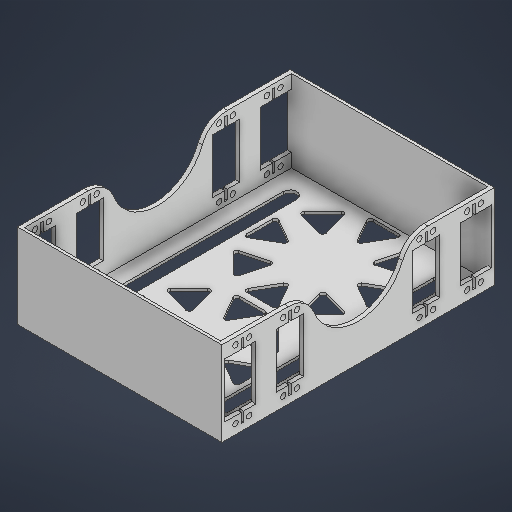
# Autodesk Inventor part: platform
Saved by Autodesk Inventor 2027.1 (Build 311270010, 270A)
## iProperties
Created: 2026-09-04
Part Number: platform
Material: Ogólny
Document SubType Name: Modeling
Designer: User
Density: 1 g/cm^3
Appearance: Domyślna
Author: User
Autodesk Inventor part; units mm, degrees
ref_plane "YZ Plane" through (0, 0, 0) normal (1, 0, 0) x (0, 1, 0)
ref_plane "XZ Plane" through (0, 0, 0) normal (0, 1, 0) x (-1, 0, 0)
ref_plane "XY Plane" through (0, 0, 0) normal (0, 0, 1) x (1, 0, 0)
sketch "Szkic1" plane through (0, 0, 0) normal (0, 1, 0) x (-1, 0, 0)
  line L0 (75, 100) -> (-75, 100)
  line L1 (-75, 100) -> (-75, -100)
  line L2 (-75, -100) -> (75, -100)
  line L3 (75, -100) -> (75, 100)
  line L4 (75, 100) -> (-75, -100) construction
  line L5 (-75, 100) -> (75, -100) construction
  line L6 (70, 95) -> (-70, 95)
  line L7 (-70, 95) -> (-70, -95)
  line L8 (-70, -95) -> (70, -95)
  line L9 (70, -95) -> (70, 95)
  line L10 (70, 95) -> (-70, -95) construction
  line L11 (-70, 95) -> (70, -95) construction
  point P0 (0, 0)
  dimension "d0" = 150
  dimension "d1" = 200
  dimension "d2" = 140
  dimension "d3" = 190
  constraints: 24 end point, 4 midpoint, 4 parallel, 2 horizontal, 2 perpendicular
  measures "d0" distance of L2.end L1.end
  measures "d1" distance of L1.end L0.end
  measures "d2" distance of L8.end L7.end
  measures "d3" distance of L7.end L6.end
extrude "Wyciągnięcie proste1" add sketch "Szkic1" against normal blind 5 contours L3 L2 L1 L0 | L9 L8 L7 L6
extrude "Wyciągnięcie proste2" add sketch "Szkic1" along normal blind 60
sketch "Szkic2" plane through (75, -5, 100) normal (1, 0, 0) x (0, 0, -1)
  line L0 (5, 5) -> (5, 65) construction
  line L1 (0, 65) -> (0, 5) construction
  line L2 (195, 5) -> (5, 5) construction
  line L3 (195, 5) -> (195, 65) construction
  line L4 (5, 5) -> (195, 5) construction
  line L5 (-69.1364, 59.5845) -> (-69.1364, 52.5845)
  line L6 (-69.1364, 52.5845) -> (-70.7364, 52.5845)
  line L7 (-70.7364, 52.5845) -> (-70.7364, 59.5845)
  line L8 (-70.7364, 59.5845) -> (-79.9364, 59.5845)
  line L9 (-79.9364, 59.5845) -> (-79.9364, 99.5845)
  line L10 (-79.9364, 99.5845) -> (-70.7364, 99.5845)
  line L11 (-70.7364, 99.5845) -> (-70.7364, 106.5845)
  line L12 (-70.7364, 106.5845) -> (-69.1364, 106.5845)
  line L13 (-69.1364, 106.5845) -> (-69.1364, 99.5845)
  line L14 (-69.1364, 99.5845) -> (-59.9364, 99.5845)
  line L15 (-59.9364, 99.5845) -> (-59.9364, 59.5845)
  line L16 (-59.9364, 59.5845) -> (-69.1364, 59.5845)
  line L17 (-117.4364, 108.0845) -> (-117.4364, 51.0845)
  line L18 (-117.4364, 51.0845) -> (-57.4364, 51.0845)
  line L19 (-57.4364, 51.0845) -> (-57.4364, 108.0845)
  line L20 (-57.4364, 108.0845) -> (-117.4364, 108.0845)
  circle A0 centre (-64.9364, 54.5845) radius 2
  circle A1 centre (-74.9364, 54.5845) radius 2
  circle A2 centre (-99.9364, 54.5845) radius 2
  circle A3 centre (-109.9364, 54.5845) radius 2
  circle A4 centre (-109.9364, 104.5845) radius 2
  circle A5 centre (-99.9364, 104.5845) radius 2
  circle A6 centre (-74.9364, 104.5845) radius 2
  circle A7 centre (-64.9364, 104.5845) radius 2
  line L21 (-105.7364, 52.5845) -> (-105.7364, 59.5845)
  line L22 (-105.7364, 59.5845) -> (-114.9364, 59.5845)
  line L23 (-114.9364, 59.5845) -> (-114.9364, 99.5845)
  line L24 (-114.9364, 99.5845) -> (-105.7364, 99.5845)
  line L25 (-105.7364, 99.5845) -> (-105.7364, 106.5845)
  line L26 (-105.7364, 106.5845) -> (-104.1364, 106.5845)
  line L27 (-104.1364, 106.5845) -> (-104.1364, 99.5845)
  line L28 (-104.1364, 99.5845) -> (-94.9364, 99.5845)
  line L29 (-94.9364, 99.5845) -> (-94.9364, 59.5845)
  line L30 (-94.9364, 59.5845) -> (-104.1364, 59.5845)
  line L31 (-104.1364, 59.5845) -> (-104.1364, 52.5845)
  line L32 (-104.1364, 52.5845) -> (-105.7364, 52.5845)
  line L33 (0, 35) -> (15, 35)
  line L34 (0, 35) -> (15, 35) construction
  line L35 (-117.4364, 79.5845) -> (-57.4364, 79.5845) construction
  line L36 (-87.4364, 108.0845) -> (-87.4364, 51.0845) construction
  line L37 (195, 35) -> (165, 35)
  circle A8 centre (10, 60) radius 2
  line L38 (15.8, 62) -> (15.8, 55)
  line L39 (14.2, 55) -> (14.2, 62)
  line L40 (14.2, 62) -> (15.8, 62)
  circle A9 centre (20, 60) radius 2
  circle A10 centre (55, 60) radius 2
  line L41 (49.2, 55) -> (49.2, 62)
  line L42 (50.8, 62) -> (50.8, 55)
  line L43 (49.2, 62) -> (50.8, 62)
  circle A11 centre (45, 60) radius 2
  line L44 (5, 55) -> (14.2, 55)
  circle A12 centre (10, 10) radius 2
  line L45 (14.2, 8) -> (14.2, 15)
  line L46 (15.8, 8) -> (14.2, 8)
  line L47 (15.8, 15) -> (15.8, 8)
  line L48 (50.8, 15) -> (50.8, 8)
  line L49 (50.8, 8) -> (49.2, 8)
  line L50 (49.2, 8) -> (49.2, 15)
  circle A13 centre (45, 10) radius 2
  line L51 (60, 15) -> (50.8, 15)
  circle A14 centre (55, 10) radius 2
  line L52 (15.8, 55) -> (25, 55)
  line L53 (40, 55) -> (49.2, 55)
  line L54 (5, 15) -> (5, 55)
  line L55 (14.2, 15) -> (5, 15)
  line L56 (25, 55) -> (25, 15)
  line L57 (50.8, 55) -> (60, 55)
  circle A15 centre (20, 10) radius 2
  line L58 (2.5, 63.5) -> (2.5, 6.5)
  line L59 (62.5, 63.5) -> (2.5, 63.5)
  line L60 (40, 15) -> (40, 55)
  line L61 (60, 55) -> (60, 15)
  line L62 (62.5, 6.5) -> (62.5, 63.5)
  line L63 (49.2, 15) -> (40, 15)
  line L64 (2.5, 6.5) -> (62.5, 6.5)
  line L65 (25, 15) -> (15.8, 15)
  line L66 (2.5, 35) -> (62.5, 35) construction
  line L67 (32.5, 63.5) -> (32.5, 6.5) construction
  line L68 (5, 55) -> (5, 63.5)
  line L69 (5, 15) -> (5, 5)
  point P0 (100, 5)
  point P1 (-104.9364, 79.5845)
  dimension "d8" = 15
  dimension "d10" = 30
  constraints: 134 end point, 16 centre point, 10 midpoint, 2 collinear, 2 horizontal, 2 point on line, 1 vertical
  measures "d8" distance of L33.start L33.end
  measures "d10" distance of L37.start L37.end
extrude "Wyciągnięcie proste3" cut sketch "Szkic2" against normal blind 60 contours L54 L44 L39 L40 L38 L52 L56 L65 L47 L46 L45 L55 | A8 | A9 | A10 | L41 L43 L42 L57 L61 L51 L48 L49 L50 L63 L60 L53 | A11 | A12 | A13 | A14 | A15
pattern_linear "Szyk prostokątny1" count 2 spacing 135 along (0, 0, -1) of "Wyciągnięcie proste3"
mirror "Odbij1" about plane through (0, 0, 0) normal (1, 0, 0) of "Wyciągnięcie proste3", "Szyk prostokątny1"
move faces "Przesuń1" translate (0, 0, 3) faces at (-23.3333, 23.3333, 95)
move faces "Przesuń2" translate (0, 0, -3) faces at (23.3333, 23.3333, -95)
sketch "Szkic3" plane through (75, -5, 100) normal (1, 0, 0) x (0, 0, -1)
  line L0 (0, 65) -> (200, 65) projected
  line L1 (0, 65) -> (200, 65)
  line L2 (100, 65) -> (100, 5)
  circle A0 centre (100, 65) radius 35
  point P0 (135, 65)
  point P1 (65, 65)
  dimension "d22" = 70
  constraints: 4 end point, 1 centre point, 1 coincident, 1 horizontal, 1 midpoint, 1 vertical
  measures "d22" diameter of A0
extrude "Wyciągnięcie proste4" cut sketch "Szkic3" against normal blind 198.25 contours L2 A0 L0 | L0 A0 L2
fillet "Zaokrąglenie1" radius 20 4 edges at (72.5, 60, 35) (72.5, 60, -35) (-72.5, 60, 35) (-72.5, 60, -35)
move faces "Przesuń3" translate (0, 3, 0) faces at (25, -5, 33.3333)
sketch "Szkic4" plane through (0, 0, 0) normal (0, 1, 0) x (1, 0, 0)
  line L0 (-70, 98) -> (-70, -98) projected
  line L1 (70, 98) -> (-70, 98)
  line L2 (-70, 98) -> (-70, -98)
  line L3 (-70, -98) -> (70, -98)
  line L4 (70, -98) -> (70, 98)
  line L5 (70, 98) -> (-70, -98) construction
  line L6 (-70, 98) -> (70, -98) construction
  line L7 (0, 0) -> (0, 25) construction
  line L8 (-1.7321, 22) -> (-11.2583, 5.5)
  line L9 (0, 25) -> (19.0526, 25) construction
  line L10 (1.7321, 22) -> (11.2583, 5.5)
  line L11 (0, 25) -> (19.0526, 25) construction
  line L12 (9.5263, 2.5) -> (-9.5263, 2.5)
  line L13 (0, 25) -> (0, 49) construction
  arc A0 (-11.2583, 5.5) -> (-9.5263, 2.5) centre (-9.5263, 4.5) ccw
  arc A1 (9.5263, 2.5) -> (11.2583, 5.5) centre (9.5263, 4.5) ccw
  arc A2 (1.7321, 22) -> (-1.7321, 22) centre (0, 21) ccw
  arc A3 (22.7983, 10.28) -> (26.1444, 9.3834) centre (24.7302, 10.7977) ccw
  line L14 (39.6166, 22.8556) -> (26.1444, 9.3834)
  line L15 (17.8671, 28.6834) -> (22.7983, 10.28)
  arc A4 (20.3166, 31.1329) -> (17.8671, 28.6834) centre (19.799, 29.201) ccw
  line L16 (34.6482, 14.3518) -> (16.9706, 32.0294) construction
  line L17 (20.3166, 31.1329) -> (38.72, 26.2017)
  line L18 (-84.1457, 34.1508) -> (153.4422, -5.4472) construction
  line L19 (14.8492, 133.1457) -> (54.4472, -104.4422) construction
  arc A5 (39.6166, 22.8556) -> (38.72, 26.2017) centre (38.2023, 24.2698) ccw
  arc A6 (43.5, 37.7417) -> (46.5, 39.4737) centre (44.5, 39.4737) ccw
  line L20 (46.5, 58.5263) -> (46.5, 39.4737)
  line L21 (27, 47.2679) -> (43.5, 37.7417)
  arc A7 (27, 50.7321) -> (27, 47.2679) centre (28, 49) ccw
  line L22 (49, 49) -> (24, 49) construction
  line L23 (27, 50.7321) -> (43.5, 60.2583)
  line L24 (-49, -21) -> (147, 119) construction
  line L25 (-49, 119) -> (147, -21) construction
  arc A8 (46.5, 58.5263) -> (43.5, 60.2583) centre (44.5, 58.5263) ccw
  arc A9 (38.72, 71.7983) -> (39.6166, 75.1444) centre (38.2023, 73.7302) ccw
  line L26 (26.1444, 88.6166) -> (39.6166, 75.1444)
  line L27 (20.3166, 66.8671) -> (38.72, 71.7983)
  arc A10 (17.8671, 69.3166) -> (20.3166, 66.8671) centre (19.799, 68.799) ccw
  line L28 (34.6482, 83.6482) -> (16.9706, 65.9706) construction
  line L29 (17.8671, 69.3166) -> (22.7983, 87.72)
  line L30 (14.8492, -35.1457) -> (54.4472, 202.4422) construction
  line L31 (-84.1457, 63.8492) -> (153.4422, 103.4472) construction
  arc A11 (26.1444, 88.6166) -> (22.7983, 87.72) centre (24.7302, 87.2023) ccw
  arc A12 (11.2583, 92.5) -> (9.5263, 95.5) centre (9.5263, 93.5) ccw
  line L32 (-9.5263, 95.5) -> (9.5263, 95.5)
  line L33 (1.7321, 76) -> (11.2583, 92.5)
  arc A13 (-1.7321, 76) -> (1.7321, 76) centre (0, 77) ccw
  line L34 (0, 98) -> (0, 73) construction
  line L35 (-1.7321, 76) -> (-11.2583, 92.5)
  line L36 (70, 0) -> (-70, 196) construction
  line L37 (-70, 0) -> (70, 196) construction
  arc A14 (-9.5263, 95.5) -> (-11.2583, 92.5) centre (-9.5263, 93.5) ccw
  arc A15 (-22.7983, 87.72) -> (-26.1444, 88.6166) centre (-24.7302, 87.2023) ccw
  line L38 (-39.6166, 75.1444) -> (-26.1444, 88.6166)
  line L39 (-17.8671, 69.3166) -> (-22.7983, 87.72)
  arc A16 (-20.3166, 66.8671) -> (-17.8671, 69.3166) centre (-19.799, 68.799) ccw
  line L40 (-34.6482, 83.6482) -> (-16.9706, 65.9706) construction
  line L41 (-20.3166, 66.8671) -> (-38.72, 71.7983)
  line L42 (84.1457, 63.8492) -> (-153.4422, 103.4472) construction
  line L43 (-14.8492, -35.1457) -> (-54.4472, 202.4422) construction
  arc A17 (-39.6166, 75.1444) -> (-38.72, 71.7983) centre (-38.2023, 73.7302) ccw
  arc A18 (-43.5, 60.2583) -> (-46.5, 58.5263) centre (-44.5, 58.5263) ccw
  line L44 (-46.5, 39.4737) -> (-46.5, 58.5263)
  line L45 (-27, 50.7321) -> (-43.5, 60.2583)
  arc A19 (-27, 47.2679) -> (-27, 50.7321) centre (-28, 49) ccw
  line L46 (-49, 49) -> (-24, 49) construction
  line L47 (-27, 47.2679) -> (-43.5, 37.7417)
  line L48 (49, 119) -> (-147, -21) construction
  line L49 (49, -21) -> (-147, 119) construction
  arc A20 (-46.5, 39.4737) -> (-43.5, 37.7417) centre (-44.5, 39.4737) ccw
  arc A21 (-38.72, 26.2017) -> (-39.6166, 22.8556) centre (-38.2023, 24.2698) ccw
  line L50 (-26.1444, 9.3834) -> (-39.6166, 22.8556)
  line L51 (-20.3166, 31.1329) -> (-38.72, 26.2017)
  arc A22 (-17.8671, 28.6834) -> (-20.3166, 31.1329) centre (-19.799, 29.201) ccw
  line L52 (-34.6482, 14.3518) -> (-16.9706, 32.0294) construction
  line L53 (-17.8671, 28.6834) -> (-22.7983, 10.28)
  line L54 (-14.8492, 133.1457) -> (-54.4472, -104.4422) construction
  line L55 (84.1457, 34.1508) -> (-153.4422, -5.4472) construction
  arc A23 (-26.1444, 9.3834) -> (-22.7983, 10.28) centre (-24.7302, 10.7977) ccw
  line L56 (-70, 0) -> (70, 0) construction
  line L57 (70, -98) -> (-70, 98) construction
  line L58 (-70, -98) -> (70, 98) construction
  line L59 (0, 0) -> (0, -25) construction
  line L60 (-1.7321, -22) -> (-11.2583, -5.5)
  line L61 (0, -25) -> (19.0526, -25) construction
  line L62 (1.7321, -22) -> (11.2583, -5.5)
  line L63 (0, -25) -> (19.0526, -25) construction
  line L64 (9.5263, -2.5) -> (-9.5263, -2.5)
  line L65 (0, -25) -> (0, -49) construction
  arc A24 (-9.5263, -2.5) -> (-11.2583, -5.5) centre (-9.5263, -4.5) ccw
  arc A25 (11.2583, -5.5) -> (9.5263, -2.5) centre (9.5263, -4.5) ccw
  arc A26 (-1.7321, -22) -> (1.7321, -22) centre (0, -21) ccw
  arc A27 (26.1444, -9.3834) -> (22.7983, -10.28) centre (24.7302, -10.7977) ccw
  line L66 (39.6166, -22.8556) -> (26.1444, -9.3834)
  line L67 (17.8671, -28.6834) -> (22.7983, -10.28)
  arc A28 (17.8671, -28.6834) -> (20.3166, -31.1329) centre (19.799, -29.201) ccw
  line L68 (34.6482, -14.3518) -> (16.9706, -32.0294) construction
  line L69 (20.3166, -31.1329) -> (38.72, -26.2017)
  line L70 (-84.1457, -34.1508) -> (153.4422, 5.4472) construction
  line L71 (14.8492, -133.1457) -> (54.4472, 104.4422) construction
  arc A29 (38.72, -26.2017) -> (39.6166, -22.8556) centre (38.2023, -24.2698) ccw
  arc A30 (46.5, -39.4737) -> (43.5, -37.7417) centre (44.5, -39.4737) ccw
  line L72 (46.5, -58.5263) -> (46.5, -39.4737)
  line L73 (27, -47.2679) -> (43.5, -37.7417)
  arc A31 (27, -47.2679) -> (27, -50.7321) centre (28, -49) ccw
  line L74 (49, -49) -> (24, -49) construction
  line L75 (27, -50.7321) -> (43.5, -60.2583)
  line L76 (-49, 21) -> (147, -119) construction
  line L77 (-49, -119) -> (147, 21) construction
  arc A32 (43.5, -60.2583) -> (46.5, -58.5263) centre (44.5, -58.5263) ccw
  arc A33 (39.6166, -75.1444) -> (38.72, -71.7983) centre (38.2023, -73.7302) ccw
  line L78 (26.1444, -88.6166) -> (39.6166, -75.1444)
  line L79 (20.3166, -66.8671) -> (38.72, -71.7983)
  arc A34 (20.3166, -66.8671) -> (17.8671, -69.3166) centre (19.799, -68.799) ccw
  line L80 (34.6482, -83.6482) -> (16.9706, -65.9706) construction
  line L81 (17.8671, -69.3166) -> (22.7983, -87.72)
  line L82 (14.8492, 35.1457) -> (54.4472, -202.4422) construction
  line L83 (-84.1457, -63.8492) -> (153.4422, -103.4472) construction
  arc A35 (22.7983, -87.72) -> (26.1444, -88.6166) centre (24.7302, -87.2023) ccw
  arc A36 (9.5263, -95.5) -> (11.2583, -92.5) centre (9.5263, -93.5) ccw
  line L84 (1.7321, -76) -> (11.2583, -92.5)
  arc A37 (1.7321, -76) -> (-1.7321, -76) centre (0, -77) ccw
  line L85 (0, -98) -> (0, -73) construction
  line L86 (-1.7321, -76) -> (-11.2583, -92.5)
  line L87 (70, 0) -> (-70, -196) construction
  line L88 (-70, 0) -> (70, -196) construction
  arc A38 (-11.2583, -92.5) -> (-9.5263, -95.5) centre (-9.5263, -93.5) ccw
  arc A39 (-26.1444, -88.6166) -> (-22.7983, -87.72) centre (-24.7302, -87.2023) ccw
  line L89 (-39.6166, -75.1444) -> (-26.1444, -88.6166)
  line L90 (-17.8671, -69.3166) -> (-22.7983, -87.72)
  arc A40 (-17.8671, -69.3166) -> (-20.3166, -66.8671) centre (-19.799, -68.799) ccw
  line L91 (-34.6482, -83.6482) -> (-16.9706, -65.9706) construction
  line L92 (-20.3166, -66.8671) -> (-38.72, -71.7983)
  line L93 (84.1457, -63.8492) -> (-153.4422, -103.4472) construction
  line L94 (-14.8492, 35.1457) -> (-54.4472, -202.4422) construction
  arc A41 (-38.72, -71.7983) -> (-39.6166, -75.1444) centre (-38.2023, -73.7302) ccw
  arc A42 (-46.5, -58.5263) -> (-43.5, -60.2583) centre (-44.5, -58.5263) ccw
  line L95 (-46.5, -39.4737) -> (-46.5, -58.5263)
  line L96 (-27, -50.7321) -> (-43.5, -60.2583)
  arc A43 (-27, -50.7321) -> (-27, -47.2679) centre (-28, -49) ccw
  line L97 (-49, -49) -> (-24, -49) construction
  line L98 (-27, -47.2679) -> (-43.5, -37.7417)
  line L99 (49, -119) -> (-147, 21) construction
  line L100 (49, 21) -> (-147, -119) construction
  arc A44 (-43.5, -37.7417) -> (-46.5, -39.4737) centre (-44.5, -39.4737) ccw
  arc A45 (-39.6166, -22.8556) -> (-38.72, -26.2017) centre (-38.2023, -24.2698) ccw
  line L101 (-26.1444, -9.3834) -> (-39.6166, -22.8556)
  line L102 (-20.3166, -31.1329) -> (-38.72, -26.2017)
  arc A46 (-20.3166, -31.1329) -> (-17.8671, -28.6834) centre (-19.799, -29.201) ccw
  line L103 (-34.6482, -14.3518) -> (-16.9706, -32.0294) construction
  line L104 (-17.8671, -28.6834) -> (-22.7983, -10.28)
  line L105 (-14.8492, -133.1457) -> (-54.4472, 104.4422) construction
  line L106 (84.1457, -34.1508) -> (-153.4422, 5.4472) construction
  arc A47 (-22.7983, -10.28) -> (-26.1444, -9.3834) centre (-24.7302, -10.7977) ccw
  line L107 (-9.5263, -95.5) -> (9.5263, -95.5)
  line L108 (-75, -100) -> (75, -100) projected
  line L109 (0, 0) -> (-70, 0)
  line L110 (-70, 0) -> (-37.0402, 0)
  line L111 (-70, 0) -> (-55, 0)
  line L112 (-55, -80) -> (-55, 80) construction
  line L113 (-50, -80) -> (-50, 80)
  line L114 (-60, 80) -> (-60, -80)
  arc A48 (-60, -80) -> (-50, -80) centre (-55, -80) ccw
  arc A49 (-50, 80) -> (-60, 80) centre (-55, 80) ccw
  line L115 (-55, 0) -> (105, 0) construction
  line L116 (70, 0) -> (55, 0)
  line L117 (55, -80) -> (55, 80) construction
  line L118 (60, -80) -> (60, 80)
  line L119 (50, 80) -> (50, -80)
  arc A50 (50, -80) -> (60, -80) centre (55, -80) ccw
  arc A51 (60, 80) -> (50, 80) centre (55, 80) ccw
  line L120 (55, 0) -> (215, 0) construction
  point P0 (12.9904, 2.5)
  point P1 (42.0661, 25.3051)
  point P2 (46.5, 61.9904)
  point P3 (23.6949, 91.0661)
  point P4 (-12.9904, 95.5)
  point P5 (-42.0661, 72.6949)
  point P6 (-46.5, 36.0096)
  point P7 (-23.6949, 6.9339)
  point P8 (12.9904, -2.5)
  point P9 (42.0661, -25.3051)
  point P10 (46.5, -61.9904)
  point P11 (23.6949, -91.0661)
  point P12 (-42.0661, -72.6949)
  point P13 (-46.5, -36.0096)
  point P14 (-23.6949, -6.9339)
  point P15 (-9.5263, -95.5)
  dimension "d30" = 120
  dimension "d31" = 60
  dimension "d32" = 95.5
  dimension "d33" = 22.5
  dimension "d34" = 24
  dimension "d35" = 2
  dimension "d38" = 360
  dimension "d40" = 15
  dimension "d41" = 80
  dimension "d42" = 90
  dimension "d43" = 10
  dimension "d44" = 15
  dimension "d45" = 80
  dimension "d46" = 90
  dimension "d47" = 10
  constraints: 242 end point, 129 symmetric about line, 104 point on circle, 66 point on line, 52 centre point, 14 tangent, 6 horizontal, 5 midpoint, 5 parallel, 4 equal length, 3 perpendicular, 2 equal radius, 2 vertical, 225 other
  measures "d30" angle of L8 L9
  measures "d31" angle of L10 L11
  measures "d32" distance between parallel lines of L1 L12
  measures "d33" vertical distance of L7.end point (12.99, 2.5)
  measures "d34" distance of L7.end L13.end
  measures "d35" radius of A0
  measures "d40" distance of L88.start L111.end
  measures "d41" distance of L111.end L112.end
  measures "d42" angle of L115 L112
  measures "d43" diameter of A49
  measures "d44" distance of L36.start L116.end
  measures "d45" distance of L116.end L117.end
  measures "d46" angle of L120 L117
  measures "d47" diameter of A51
extrude "Wyciągnięcie proste5" cut sketch "Szkic4" against normal blind 2 contours A2 L10 A1 L12 A0 L8 | L15 A4 L17 A5 L14 A3 | L21 A7 L23 A8 L20 A6 | L27 A10 L29 A11 L26 A9 | L33 A13 L35 A14 L32 A12 | L39 A16 L41 A17 L38 A15 | L45 A19 L47 A20 L44 A18 | L51 A22 L53 A23 L50 A21 | L60 A24 L64 A25 L62 A26 | L66 A29 L69 A28 L67 A27 | L72 A32 L75 A31 L73 A30 | L78 A35 L81 A34 L79 A33 | L107 A38 L86 A37 L84 A36 | L89 A41 L92 A40 L90 A39 | L95 A44 L98 A43 L96 A42 | L101 A47 L104 A46 L102 A45 | L113 A48 L114 L109 | L109 L114 A49 L113 | A50 L119 A51 L118
move faces "Przesuń4" translate (-2, 0, 0) faces at (-70, 10.8517, 1.2688)
move faces "Przesuń5" translate (2, 0, 0) faces at (70, 10.8517, 1.2688)
